Autodesk Inventor part; units mm, degrees
(part 2 of 3)
  measures "d37" diameter of A260
extrude "Extrusion3" add sketch "Sketch3" along normal blind 7.1 contours A0 | A211 | A196 L243 A245 | L243 A245 A196 | A159 | A208 | L220 A246 L224 A185 | A185 L224 A246 L220 | A206 | L219 A248 L216 A180 | A180 L216 A248 L219 | A151 | A153 | A189 | A207 | A213 | A218 | A221 | A222
extrude "Extrusion4" add sketch "Sketch3" along normal blind 2 contours A260 | A257 | A258 | A259
mirror "Mirror1" about plane through (0, 0, 0) normal (1, 0, 0) of "Extrusion4"
extrude "Extrusion5" add sketch "Sketch1" against normal up to surface (3 mm away) contours A10 L72 | L72 A10 | A75 | A27 | A76 | A77 L70 A15 L26 | L26 A15 L70 A77 | L26 L70 A15 | A15 L70 L26 | A78 L28 A12 L69 | L69 A12 L28 A78 | L69 L28 A12 | A12 L28 L69
mirror "Mirror2" about plane through (0, 0, 0) normal (1, 0, 0) of "Extrusion5"
sketch "Sketch4" plane through (0, 5, 0) normal (0, 1, 0) x (1, 0, 0)
  circle A0 centre (0, 0) radius 5.5
  dimension "d46" = 11
  constraints: 1 centre point, 1 coincident
  measures "d46" diameter of A0
extrude "Extrusion6" cut sketch "Sketch4" against normal blind 15
sketch "Sketch5" plane through (0, 5, 0) normal (0, 1, 0) x (1, 0, 0)
  arc A0 (19.2671, 3.2712) -> (23.1562, 4.8822) centre (19.2671, 8.7712) ccw projected
  line L0 (23.1562, 4.8822) -> (40.8632, 22.5892) projected
  circle A1 centre (17.1458, 27.8631) radius 5.5 projected
  circle A2 centre (17.1458, 27.8631) radius 5.5 projected
  arc A3 (23.1562, 4.8822) -> (19.2671, 3.2712) centre (19.2671, 8.7712) ccw projected
  line L1 (23.1562, 4.8822) -> (31.6415, 13.3674) projected
  circle A4 centre (27.7524, 17.2565) radius 5.5 projected
  circle A5 centre (27.7524, 17.2565) radius 5.5 projected
  line L2 (31.6415, 13.3674) -> (40.8632, 22.5892) projected
  line L3 (40.8632, 22.5892) -> (22.4784, 40.9739) projected
  line L4 (40.8632, 22.5892) -> (22.4784, 40.9739) projected
  line L5 (22.4784, 40.9739) -> (13.2567, 31.7522) projected
  line L6 (22.4784, 40.9739) -> (4.7714, 23.2669) projected
  circle A6 centre (8.6605, -19.0931) radius 2.5 projected
  circle A7 centre (8.6605, -19.0931) radius 1.5 projected
  circle A8 centre (19.2671, -8.4864) radius 1.5 projected
  circle A9 centre (19.2671, -8.4864) radius 1.5 projected
  circle A10 centre (19.2671, -8.4864) radius 1.5 projected
  circle A11 centre (19.2671, -8.4864) radius 2.5 projected
  circle A12 centre (19.2671, -8.4864) radius 2.5 projected
  circle A13 centre (19.2671, -8.4864) radius 2.5 projected
  circle A14 centre (19.2671, -8.4864) radius 3 projected
  circle A15 centre (19.2671, -8.4864) radius 5.5 projected
  circle A16 centre (19.2671, -8.4864) radius 3 projected
  circle A17 centre (19.2671, -8.4864) radius 3 projected
  circle A18 centre (19.2671, -8.4864) radius 2.5 projected
  circle A19 centre (19.2671, -8.4864) radius 3 projected
  circle A20 centre (19.2671, -8.4864) radius 3 projected
  circle A21 centre (8.6605, -19.0931) radius 1.5 projected
  circle A22 centre (8.6605, -19.0931) radius 1.5 projected
  circle A23 centre (8.6605, -19.0931) radius 1.5 projected
  circle A24 centre (8.6605, -19.0931) radius 1.5 projected
  circle A25 centre (8.6605, -19.0931) radius 2.5 projected
  circle A26 centre (8.6605, -19.0931) radius 1.5 projected
  circle A27 centre (8.6605, -19.0931) radius 2.5 projected
  circle A28 centre (8.6605, -19.0931) radius 2.5 projected
  circle A29 centre (8.6605, -19.0931) radius 2.5 projected
  circle A30 centre (8.6605, -19.0931) radius 3 projected
  circle A31 centre (8.6605, -19.0931) radius 3 projected
  circle A32 centre (8.6605, -19.0931) radius 2.5 projected
  circle A33 centre (8.6605, -19.0931) radius 3 projected
  circle A34 centre (8.6605, -19.0931) radius 3 projected
  circle A35 centre (8.6605, -19.0931) radius 3 projected
  circle A36 centre (8.6605, -19.0931) radius 5.5 projected
  circle A37 centre (8.6605, -19.0931) radius 5.5 projected
  arc A38 (3.1605, -19.0931) -> (4.7714, -22.9821) centre (8.6605, -19.0931) ccw projected
  arc A39 (4.7714, -22.9821) -> (3.1605, -19.0931) centre (8.6605, -19.0931) ccw projected
  line L7 (3.1605, -5.8386) -> (3.1605, -19.0931) projected
  line L8 (3.1605, -5.8386) -> (3.1605, -19.0931) projected
  circle A40 centre (19.2671, -8.4864) radius 1.5 projected
  arc A41 (23.1562, -4.5974) -> (19.2671, -2.9864) centre (19.2671, -8.4864) ccw projected
  line L9 (19.2671, -2.9864) -> (6.0127, -2.9864) projected
  arc A42 (6.0127, -2.9864) -> (6.0127, 3.2712) centre (0.0316, 0.1424) ccw projected
  line L10 (6.0127, 3.2712) -> (19.2671, 3.2712) projected
  arc A43 (3.1605, 6.1234) -> (-3.0972, 6.1234) centre (0.0316, 0.1424) ccw projected
  line L11 (6.0127, 3.2712) -> (19.2671, 3.2712) projected
  arc A44 (3.1605, 6.1234) -> (-3.0972, 6.1234) centre (0.0316, 0.1424) ccw projected
  arc A45 (3.1605, 6.1234) -> (-3.0972, 6.1234) centre (0.0316, 0.1424) ccw projected
  arc A46 (3.1605, 6.1234) -> (-3.0972, 6.1234) centre (0.0316, 0.1424) ccw projected
  arc A47 (6.0127, -2.9864) -> (6.0127, 3.2712) centre (0.0316, 0.1424) ccw projected
  line L12 (19.2671, -2.9864) -> (6.0127, -2.9864) projected
  arc A48 (6.0127, -2.9864) -> (6.0127, 3.2712) centre (0.0316, 0.1424) ccw projected
  arc A49 (6.0127, -2.9864) -> (6.0127, 3.2712) centre (0.0316, 0.1424) ccw projected
  arc A50 (19.2671, -2.9864) -> (23.1562, -4.5974) centre (19.2671, -8.4864) ccw projected
  arc A51 (-3.0972, -5.8386) -> (3.1605, -5.8386) centre (0.0316, 0.1424) ccw projected
  arc A52 (-3.0972, -5.8386) -> (3.1605, -5.8386) centre (0.0316, 0.1424) ccw projected
  circle A53 centre (0, 0) radius 5.5 projected
  line L13 (3.1605, -5.8386) -> (3.1605, -19.0931) projected
  arc A54 (3.1605, -19.0931) -> (4.7714, -22.9821) centre (8.6605, -19.0931) ccw projected
  line L14 (-3.0972, -19.0931) -> (-3.0972, -5.8386) projected
  circle A55 centre (0, 0) radius 5.5 projected
  circle A56 centre (17.1458, -27.5783) radius 2.5 projected
  circle A57 centre (17.1458, -27.5783) radius 1.5 projected
  circle A58 centre (17.1458, -27.5783) radius 1.5 projected
  circle A59 centre (17.1458, -27.5783) radius 2.5 projected
  circle A60 centre (17.1458, -27.5783) radius 3 projected
  line L15 (22.4651, -26.1801) -> (18.544, -22.259) projected
  line L16 (18.544, -22.259) -> (22.4651, -26.1801) projected
  arc A61 (18.544, -22.259) -> (13.2567, -31.4674) centre (17.1458, -27.5783) ccw projected
  arc A62 (18.544, -22.259) -> (22.4651, -26.1801) centre (17.1458, -27.5783) ccw projected
  arc A63 (13.2567, -31.4674) -> (22.4651, -26.1801) centre (17.1458, -27.5783) ccw projected
  circle A64 centre (17.1458, -27.5783) radius 3 projected
  line L17 (18.544, -22.259) -> (22.4651, -26.1801) projected
  arc A65 (18.544, -22.259) -> (22.4651, -26.1801) centre (17.1458, -27.5783) ccw projected
  circle A66 centre (17.1458, -27.5783) radius 1.5 projected
  circle A67 centre (17.1458, -27.5783) radius 1.5 projected
  circle A68 centre (17.1458, -27.5783) radius 1.5 projected
  circle A69 centre (17.1458, -27.5783) radius 2.5 projected
  circle A70 centre (17.1458, -27.5783) radius 2.5 projected
  circle A71 centre (17.1458, -27.5783) radius 3 projected
  circle A72 centre (17.1458, -27.5783) radius 3 projected
  circle A73 centre (17.1458, -27.5783) radius 3 projected
  circle A74 centre (17.1458, -27.5783) radius 2.5 projected
  circle A75 centre (17.1458, -27.5783) radius 2.5 projected
  circle A76 centre (17.1458, -27.5783) radius 1.5 projected
  line L18 (3.1605, -5.8386) -> (3.1605, -19.0931) projected
  arc A77 (4.7714, -22.9821) -> (3.1605, -19.0931) centre (8.6605, -19.0931) ccw projected
  line L19 (4.7714, -22.9821) -> (13.2567, -31.4674) projected
  line L20 (31.6415, -13.0826) -> (23.1562, -4.5974) projected
  circle A78 centre (19.2671, -8.4864) radius 5.5 projected
  line L21 (22.4651, -26.1801) -> (18.544, -22.259) projected
  line L22 (22.4331, -18.3699) -> (26.3542, -22.291) projected
  arc A79 (18.544, -22.259) -> (13.2567, -31.4674) centre (17.1458, -27.5783) ccw projected
  arc A80 (31.6415, -13.0826) -> (22.4331, -18.3699) centre (27.7524, -16.9717) ccw projected
  arc A81 (26.3542, -22.291) -> (31.6415, -13.0826) centre (27.7524, -16.9717) ccw projected
  arc A82 (13.2567, -31.4674) -> (22.4651, -26.1801) centre (17.1458, -27.5783) ccw projected
  circle A83 centre (8.6605, -19.0931) radius 5.5 projected
  arc A84 (4.7714, 23.2669) -> (3.1605, 19.3778) centre (8.6605, 19.3778) ccw projected
  line L23 (3.1605, 19.3778) -> (3.1605, 6.1234) projected
  line L24 (-3.0972, 6.1234) -> (-3.0972, 19.3778) projected
  arc A85 (-3.0972, 19.3778) -> (-4.7081, 23.2669) centre (-8.5972, 19.3778) ccw projected
  circle A86 centre (-8.5972, 19.3778) radius 1.5 projected
  circle A87 centre (-8.5972, 19.3778) radius 2.5 projected
  arc A88 (-8.6288, 16.878) -> (-8.6288, 21.8776) centre (-8.5972, 19.3778) ccw projected
  circle A89 centre (-8.6605, 19.3778) radius 3 projected
  arc A90 (-8.6288, 21.8776) -> (-8.6288, 16.878) centre (-8.6605, 19.3778) ccw projected
  arc A91 (-3.0972, -5.8386) -> (3.1605, -5.8386) centre (0.0316, 0.1424) ccw projected
  arc A92 (-3.0972, -5.8386) -> (3.1605, -5.8386) centre (0.0316, 0.1424) ccw projected
  circle A93 centre (-8.5972, 19.3778) radius 1.5 projected
  arc A94 (-8.6288, 21.8776) -> (-8.6288, 16.878) centre (-8.6605, 19.3778) ccw projected
  arc A95 (-8.6288, 21.8776) -> (-8.6288, 16.878) centre (-8.5972, 19.3778) ccw projected
  arc A96 (-8.6288, 21.8776) -> (-8.6288, 16.878) centre (-8.6605, 19.3778) ccw projected
  arc A97 (-8.6288, 21.8776) -> (-8.6288, 16.878) centre (-8.6605, 19.3778) ccw projected
  circle A98 centre (-8.5972, 19.3778) radius 5.5 projected
  circle A99 centre (-8.6605, 19.3778) radius 3 projected
  arc A100 (-8.6288, 16.878) -> (-8.6288, 21.8776) centre (-8.5972, 19.3778) ccw projected
  arc A101 (-8.6288, 21.8776) -> (-8.6288, 16.878) centre (-8.6605, 19.3778) ccw projected
  circle A102 centre (-8.6605, 19.3778) radius 3 projected
  circle A103 centre (-8.6605, 19.3778) radius 3 projected
  circle A104 centre (-8.6605, 19.3778) radius 3 projected
  circle A105 centre (-8.5972, 19.3778) radius 2.5 projected
  circle A106 centre (-8.5972, 19.3778) radius 1.5 projected
  arc A107 (-8.6288, 16.878) -> (-8.6288, 21.8776) centre (-8.5972, 19.3778) ccw projected
  arc A108 (-8.6288, 21.8776) -> (-8.6288, 16.878) centre (-8.5972, 19.3778) ccw projected
  circle A109 centre (-8.5972, 19.3778) radius 2.5 projected
  circle A110 centre (0, 0) radius 5.5 projected
  circle A111 centre (0, 0) radius 5.5 projected
  circle A112 centre (-8.5972, 19.3778) radius 1.5 projected
  circle A113 centre (-8.5972, 19.3778) radius 1.5 projected
  arc A114 (-19.2354, 11.271) -> (-19.2354, 6.2714) centre (-19.2038, 8.7712) ccw projected
  line L25 (13.2567, -31.4674) -> (22.4784, -40.6891) projected
  line L26 (22.4784, -40.6891) -> (40.8632, -22.3044) projected
  line L27 (40.8632, -22.3044) -> (31.6415, -13.0826) projected
  line L28 (4.7714, -22.9821) -> (22.4784, -40.6891) projected
  line L29 (22.4784, -40.6891) -> (40.8632, -22.3044) projected
  line L30 (40.8632, -22.3044) -> (23.1562, -4.5974) projected
  arc A115 (18.544, -22.259) -> (22.4651, -26.1801) centre (17.1458, -27.5783) ccw projected
  line L31 (18.544, -22.259) -> (22.4651, -26.1801) projected
  line L32 (26.3542, -22.291) -> (22.4331, -18.3699) projected
  arc A116 (26.3542, -22.291) -> (22.4331, -18.3699) centre (27.7524, -16.9717) ccw projected
  line L33 (19.2671, -2.9864) -> (6.0127, -2.9864) projected
  line L34 (19.2671, -2.9864) -> (6.0127, -2.9864) projected
  circle A117 centre (8.6605, -19.0931) radius 3 projected
  circle A118 centre (19.2671, -8.4864) radius 5.5 projected
  arc A119 (23.1562, -4.5974) -> (19.2671, -2.9864) centre (19.2671, -8.4864) ccw projected
  arc A120 (19.2671, -2.9864) -> (23.1562, -4.5974) centre (19.2671, -8.4864) ccw projected
  circle A121 centre (27.7524, -16.9717) radius 3 projected
  circle A122 centre (17.1458, -27.5783) radius 3 projected
  line L35 (4.7714, -22.9821) -> (13.2567, -31.4674) projected
  line L36 (13.2567, -31.4674) -> (22.4784, -40.6891) projected
  line L37 (4.7714, -22.9821) -> (22.4784, -40.6891) projected
  line L38 (40.8632, -22.3044) -> (31.6415, -13.0826) projected
  line L39 (31.6415, -13.0826) -> (23.1562, -4.5974) projected
  line L40 (40.8632, -22.3044) -> (23.1562, -4.5974) projected
  line L41 (22.4784, -40.6891) -> (40.8632, -22.3044) projected
  line L42 (22.4784, -40.6891) -> (40.8632, -22.3044) projected
  circle A123 centre (19.2671, -8.4864) radius 3 projected
  line L43 (13.2567, 31.7522) -> (4.7714, 23.2669) projected
  line L44 (3.1605, 19.3778) -> (3.1605, 6.1234) projected
  arc A124 (3.1605, 19.3778) -> (4.7714, 23.2669) centre (8.6605, 19.3778) ccw projected
  circle A125 centre (0, 0) radius 5.5 projected
  line L45 (4.7714, -22.9821) -> (22.4784, -40.6891) projected
  line L46 (22.4784, -40.6891) -> (40.8632, -22.3044) projected
  line L47 (40.8632, -22.3044) -> (23.1562, -4.5974) projected
  arc A126 (23.1562, -4.5974) -> (19.2671, -2.9864) centre (19.2671, -8.4864) ccw projected
  line L48 (19.2671, -2.9864) -> (6.0127, -2.9864) projected
  arc A127 (6.0127, -2.9864) -> (6.0127, 3.2712) centre (0.0316, 0.1424) ccw projected
  line L49 (6.0127, 3.2712) -> (19.2671, 3.2712) projected
  arc A128 (19.2671, 3.2712) -> (23.1562, 4.8822) centre (19.2671, 8.7712) ccw projected
  line L50 (23.1562, 4.8822) -> (40.8632, 22.5892) projected
  line L51 (40.8632, 22.5892) -> (22.4784, 40.9739) projected
  line L52 (22.4784, 40.9739) -> (4.7714, 23.2669) projected
  arc A129 (4.7714, 23.2669) -> (3.1605, 19.3778) centre (8.6605, 19.3778) ccw projected
  line L53 (3.1605, 19.3778) -> (3.1605, 6.1234) projected
  arc A130 (3.1605, 6.1234) -> (-3.0972, 6.1234) centre (0.0316, 0.1424) ccw projected
  line L54 (-3.0972, 6.1234) -> (-3.0972, 19.3778) projected
  arc A131 (-3.0972, 19.3778) -> (-4.7081, 23.2669) centre (-8.5972, 19.3778) ccw projected
  line L55 (-4.7081, 23.2669) -> (-22.4151, 40.9739) projected
  line L56 (-22.4151, 40.9739) -> (-40.7999, 22.5892) projected
  line L57 (-40.7999, 22.5892) -> (-23.0929, 4.8822) projected
  arc A132 (-23.0929, 4.8822) -> (-19.2038, 3.2712) centre (-19.2038, 8.7712) ccw projected
  line L58 (-19.2038, 3.2712) -> (-5.9494, 3.2712) projected
  arc A133 (-5.9494, 3.2712) -> (-5.9494, -2.9864) centre (0.0316, 0.1424) ccw projected
  line L59 (-5.9494, -2.9864) -> (-19.2038, -2.9864) projected
  arc A134 (-19.2038, -2.9864) -> (-23.0929, -4.5974) centre (-19.2038, -8.4864) ccw projected
  line L60 (-23.0929, -4.5974) -> (-40.7999, -22.3044) projected
  line L61 (-40.7999, -22.3044) -> (-22.4151, -40.6891) projected
  line L62 (-22.4151, -40.6891) -> (-4.7081, -22.9821) projected
  arc A135 (-4.7081, -22.9821) -> (-3.0972, -19.0931) centre (-8.5972, -19.0931) ccw projected
  line L63 (-3.0972, -19.0931) -> (-3.0972, -5.8386) projected
  arc A136 (-3.0972, -5.8386) -> (3.1605, -5.8386) centre (0.0316, 0.1424) ccw projected
  line L64 (3.1605, -5.8386) -> (3.1605, -19.0931) projected
  arc A137 (3.1605, -19.0931) -> (4.7714, -22.9821) centre (8.6605, -19.0931) ccw projected
  circle A138 centre (0, 0) radius 5.5 projected
  arc A139 (23.1562, 4.8822) -> (19.2671, 3.2712) centre (19.2671, 8.7712) ccw projected
  line L65 (6.0127, 3.2712) -> (19.2671, 3.2712) projected
  arc A140 (6.0127, -2.9864) -> (6.0127, 3.2712) centre (0.0316, 0.1424) ccw projected
  line L66 (19.2671, -2.9864) -> (6.0127, -2.9864) projected
  arc A141 (19.2671, -2.9864) -> (23.1562, -4.5974) centre (19.2671, -8.4864) ccw projected
  line L67 (31.6415, -13.0826) -> (23.1562, -4.5974) projected
  arc A142 (31.6415, -13.0826) -> (22.4331, -18.3699) centre (27.7524, -16.9717) ccw projected
  line L68 (22.4331, -18.3699) -> (26.3542, -22.291) projected
  arc A143 (26.3542, -22.291) -> (31.6415, -13.0826) centre (27.7524, -16.9717) ccw projected
  line L69 (40.8632, -22.3044) -> (31.6415, -13.0826) projected
  line L70 (22.4784, -40.6891) -> (40.8632, -22.3044) projected
  line L71 (13.2567, -31.4674) -> (22.4784, -40.6891) projected
  arc A144 (13.2567, -31.4674) -> (22.4651, -26.1801) centre (17.1458, -27.5783) ccw projected
  line L72 (22.4651, -26.1801) -> (18.544, -22.259) projected
  arc A145 (18.544, -22.259) -> (13.2567, -31.4674) centre (17.1458, -27.5783) ccw projected
  line L73 (4.7714, -22.9821) -> (13.2567, -31.4674) projected
  arc A146 (4.7714, -22.9821) -> (3.1605, -19.0931) centre (8.6605, -19.0931) ccw projected
  line L74 (3.1605, -5.8386) -> (3.1605, -19.0931) projected
  arc A147 (-3.0972, -5.8386) -> (3.1605, -5.8386) centre (0.0316, 0.1424) ccw projected
  line L75 (-3.0972, -19.0931) -> (-3.0972, -5.8386) projected
  arc A148 (-3.0972, -19.0931) -> (-4.7081, -22.9821) centre (-8.5972, -19.0931) ccw projected
  line L76 (-13.1934, -31.4674) -> (-4.7081, -22.9821) projected
  circle A149 centre (-17.0825, -27.5783) radius 5.5 projected
  line L77 (-22.4151, -40.6891) -> (-13.1934, -31.4674) projected
  line L78 (-40.7999, -22.3044) -> (-22.4151, -40.6891) projected
  line L79 (-31.5782, -13.0826) -> (-40.7999, -22.3044) projected
  circle A150 centre (-27.6891, -16.9717) radius 5.5 projected
  line L80 (-23.0929, -4.5974) -> (-31.5782, -13.0826) projected
  arc A151 (-23.0929, -4.5974) -> (-19.2038, -2.9864) centre (-19.2038, -8.4864) ccw projected
  line L81 (-5.9494, -2.9864) -> (-19.2038, -2.9864) projected
  arc A152 (-5.9494, 3.2712) -> (-5.9494, -2.9864) centre (0.0316, 0.1424) ccw projected
  line L82 (-19.2038, 3.2712) -> (-5.9494, 3.2712) projected
  arc A153 (-19.2038, 3.2712) -> (-23.0929, 4.8822) centre (-19.2038, 8.7712) ccw projected
  line L83 (-31.5782, 13.3674) -> (-23.0929, 4.8822) projected
  circle A154 centre (-27.6891, 17.2565) radius 5.5 projected
  line L84 (-40.7999, 22.5892) -> (-31.5782, 13.3674) projected
  line L85 (-22.4151, 40.9739) -> (-40.7999, 22.5892) projected
  line L86 (-13.1934, 31.7522) -> (-22.4151, 40.9739) projected
  circle A155 centre (-17.0825, 27.8631) radius 5.5 projected
  line L87 (-4.7081, 23.2669) -> (-13.1934, 31.7522) projected
  arc A156 (-4.7081, 23.2669) -> (-3.0972, 19.3778) centre (-8.5972, 19.3778) ccw projected
  line L88 (-3.0972, 6.1234) -> (-3.0972, 19.3778) projected
  arc A157 (3.1605, 6.1234) -> (-3.0972, 6.1234) centre (0.0316, 0.1424) ccw projected
  line L89 (3.1605, 19.3778) -> (3.1605, 6.1234) projected
  arc A158 (3.1605, 19.3778) -> (4.7714, 23.2669) centre (8.6605, 19.3778) ccw projected
  line L90 (13.2567, 31.7522) -> (4.7714, 23.2669) projected
  circle A159 centre (17.1458, 27.8631) radius 5.5 projected
  line L91 (22.4784, 40.9739) -> (13.2567, 31.7522) projected
  line L92 (40.8632, 22.5892) -> (22.4784, 40.9739) projected
  line L93 (31.6415, 13.3674) -> (40.8632, 22.5892) projected
  circle A160 centre (27.7524, 17.2565) radius 5.5 projected
  line L94 (23.1562, 4.8822) -> (31.6415, 13.3674) projected
  arc A161 (-4.7081, -22.9821) -> (-3.0972, -19.0931) centre (-8.5972, -19.0931) ccw projected
  arc A162 (-5.9494, 3.2712) -> (-5.9494, -2.9864) centre (0.0316, 0.1424) ccw projected
  line L95 (-4.7081, 23.2669) -> (-22.4151, 40.9739) projected
  arc A163 (-23.0929, 4.8822) -> (-19.2038, 3.2712) centre (-19.2038, 8.7712) ccw projected
  line L96 (-5.9494, -2.9864) -> (-19.2038, -2.9864) projected
  arc A164 (-19.2038, -2.9864) -> (-23.0929, -4.5974) centre (-19.2038, -8.4864) ccw projected
  line L97 (-22.4151, 40.9739) -> (-40.7999, 22.5892) projected
  line L98 (-40.7999, 22.5892) -> (-23.0929, 4.8822) projected
  line L99 (-19.2038, 3.2712) -> (-5.9494, 3.2712) projected
  arc A165 (-4.7081, 23.2669) -> (-3.0972, 19.3778) centre (-8.5972, 19.3778) ccw projected
  line L100 (-4.7081, 23.2669) -> (-13.1934, 31.7522) projected
  circle A166 centre (-19.2038, 8.7712) radius 1.5 projected
  circle A167 centre (-8.5972, 19.3778) radius 1.5 projected
  circle A168 centre (-19.2671, 8.7712) radius 3 projected
  circle A169 centre (-8.6605, 19.3778) radius 3 projected
  circle A170 centre (-8.5972, 19.3778) radius 5.5 projected
  circle A171 centre (-19.2038, 8.7712) radius 5.5 projected
  circle A172 centre (-17.0825, 27.8631) radius 1.5 projected
  circle A173 centre (-17.0825, 27.8631) radius 5.5 projected
  circle A174 centre (-27.8428, 17.2565) radius 1.5 projected
  arc A175 (-19.2354, 11.271) -> (-19.2354, 6.2714) centre (-19.2671, 8.7712) ccw projected
  circle A176 centre (-27.8428, 17.2565) radius 1.5 projected
  circle A177 centre (-17.0825, 27.8631) radius 1.5 projected
  circle A178 centre (-17.0825, 27.8631) radius 2.5 projected
  arc A179 (-17.1141, 30.3629) -> (-17.1141, 25.3633) centre (-17.0825, 27.8631) ccw projected
  circle A180 centre (-27.6891, 17.2565) radius 2.5 projected
  arc A181 (-27.7207, 19.7563) -> (-27.7207, 14.7567) centre (-27.6891, 17.2565) ccw projected
  arc A182 (-17.1141, 25.3633) -> (-17.1141, 30.3629) centre (-17.0825, 27.8631) ccw projected
  circle A183 centre (-17.1458, 27.8631) radius 3 projected
  circle A184 centre (-17.1458, 27.8631) radius 3 projected
  arc A185 (-17.1141, 30.3629) -> (-17.1141, 25.3633) centre (-17.1458, 27.8631) ccw projected
  arc A186 (-17.1141, 30.3629) -> (-17.1141, 25.3633) centre (-17.1458, 27.8631) ccw projected
  arc A187 (-27.7207, 14.7567) -> (-27.7207, 19.7563) centre (-27.6891, 17.2565) ccw projected
  circle A188 centre (-27.8428, 17.2565) radius 1.5 projected
  circle A189 centre (-27.8428, 17.2565) radius 1.5 projected
  circle A190 centre (-27.8428, 17.2565) radius 1.5 projected
  arc A191 (-17.1141, 30.3629) -> (-17.1141, 25.3633) centre (-17.1458, 27.8631) ccw projected
  arc A192 (-17.1141, 30.3629) -> (-17.1141, 25.3633) centre (-17.1458, 27.8631) ccw projected
  arc A193 (-17.1141, 30.3629) -> (-17.1141, 25.3633) centre (-17.1458, 27.8631) ccw projected
  arc A194 (-17.1141, 30.3629) -> (-17.1141, 25.3633) centre (-17.0825, 27.8631) ccw projected
  circle A195 centre (-17.0825, 27.8631) radius 1.5 projected
  circle A196 centre (-17.0825, 27.8631) radius 1.5 projected
  circle A197 centre (-17.0825, 27.8631) radius 1.5 projected
  arc A198 (-17.1141, 25.3633) -> (-17.1141, 30.3629) centre (-17.0825, 27.8631) ccw projected
  arc A199 (-17.1141, 30.3629) -> (-17.1141, 25.3633) centre (-17.1458, 27.8631) ccw projected
  circle A200 centre (-17.1458, 27.8631) radius 3 projected
  circle A201 centre (-17.1458, 27.8631) radius 3 projected
  circle A202 centre (-17.1458, 27.8631) radius 3 projected
  circle A203 centre (-17.0825, 27.8631) radius 5.5 projected
  circle A204 centre (-17.0825, 27.8631) radius 5.5 projected
  circle A205 centre (-17.0825, 27.8631) radius 5.5 projected
  circle A206 centre (-17.1458, 27.8631) radius 3 projected
  circle A207 centre (-17.0825, 27.8631) radius 2.5 projected
  circle A208 centre (-17.0825, 27.8631) radius 1.5 projected
  arc A209 (-17.1141, 25.3633) -> (-17.1141, 30.3629) centre (-17.0825, 27.8631) ccw projected
  arc A210 (-17.1141, 30.3629) -> (-17.1141, 25.3633) centre (-17.0825, 27.8631) ccw projected
  circle A211 centre (-17.0825, 27.8631) radius 2.5 projected
  arc A212 (-27.7207, 14.7567) -> (-27.7207, 19.7563) centre (-27.6891, 17.2565) ccw projected
  arc A213 (-27.7207, 19.7563) -> (-27.7207, 14.7567) centre (-27.6891, 17.2565) ccw projected
  circle A214 centre (-27.6891, 17.2565) radius 2.5 projected
  line L101 (-13.1934, 31.7522) -> (-22.4151, 40.9739) projected
  line L102 (-22.4151, 40.9739) -> (-40.7999, 22.5892) projected
  line L103 (-40.7999, 22.5892) -> (-31.5782, 13.3674) projected
  line L104 (-19.2038, 3.2712) -> (-5.9494, 3.2712) projected
  line L105 (-19.2038, 3.2712) -> (-5.9494, 3.2712) projected
  line L106 (-3.0972, 6.1234) -> (-3.0972, 19.3778) projected
  line L107 (-3.0972, 6.1234) -> (-3.0972, 19.3778) projected
  circle A215 centre (-19.2038, 8.7712) radius 5.5 projected
  arc A216 (-23.0929, 4.8822) -> (-19.2038, 3.2712) centre (-19.2038, 8.7712) ccw projected
  arc A217 (-19.2038, 3.2712) -> (-23.0929, 4.8822) centre (-19.2038, 8.7712) ccw projected
  circle A218 centre (-8.5972, 19.3778) radius 5.5 projected
  arc A219 (-3.0972, 19.3778) -> (-4.7081, 23.2669) centre (-8.5972, 19.3778) ccw projected
  arc A220 (-4.7081, 23.2669) -> (-3.0972, 19.3778) centre (-8.5972, 19.3778) ccw projected
  circle A221 centre (-27.7524, 17.2565) radius 3 projected
  line L108 (-4.7081, 23.2669) -> (-13.1934, 31.7522) projected
  line L109 (-13.1934, 31.7522) -> (-22.4151, 40.9739) projected
  line L110 (-4.7081, 23.2669) -> (-22.4151, 40.9739) projected
  line L111 (-40.7999, 22.5892) -> (-31.5782, 13.3674) projected
  line L112 (-31.5782, 13.3674) -> (-23.0929, 4.8822) projected
  line L113 (-40.7999, 22.5892) -> (-23.0929, 4.8822) projected
  line L114 (-22.4151, 40.9739) -> (-40.7999, 22.5892) projected
  line L115 (-22.4151, 40.9739) -> (-40.7999, 22.5892) projected
  arc A222 (-27.7207, 19.7563) -> (-27.7207, 14.7567) centre (-27.7524, 17.2565) ccw projected
  arc A223 (-8.6288, 21.8776) -> (-8.6288, 16.878) centre (-8.6605, 19.3778) ccw projected
  circle A224 centre (-27.6891, 17.2565) radius 5.5 projected
  circle A225 centre (-17.0825, 27.8631) radius 5.5 projected
  arc A226 (-8.6288, 21.8776) -> (-8.6288, 16.878) centre (-8.5972, 19.3778) ccw projected
  circle A227 centre (-27.6891, 17.2565) radius 2.5 projected
  circle A228 centre (-27.8428, 17.2565) radius 1.5 projected
  circle A229 centre (-19.2038, 8.7712) radius 1.5 projected
  circle A230 centre (-19.2038, 8.7712) radius 2.5 projected
  arc A231 (-19.2354, 6.2714) -> (-19.2354, 11.271) centre (-19.2038, 8.7712) ccw projected
  circle A232 centre (-19.2671, 8.7712) radius 3 projected
  arc A233 (-19.2354, 11.271) -> (-19.2354, 6.2714) centre (-19.2671, 8.7712) ccw projected
  arc A234 (-27.7207, 19.7563) -> (-27.7207, 14.7567) centre (-27.7524, 17.2565) ccw projected
  arc A235 (-27.7207, 19.7563) -> (-27.7207, 14.7567) centre (-27.6891, 17.2565) ccw projected
  arc A236 (-27.7207, 19.7563) -> (-27.7207, 14.7567) centre (-27.7524, 17.2565) ccw projected
  arc A237 (-27.7207, 19.7563) -> (-27.7207, 14.7567) centre (-27.7524, 17.2565) ccw projected
  circle A238 centre (-27.7524, 17.2565) radius 3 projected
  arc A239 (-27.7207, 14.7567) -> (-27.7207, 19.7563) centre (-27.6891, 17.2565) ccw projected
  arc A240 (-27.7207, 19.7563) -> (-27.7207, 14.7567) centre (-27.7524, 17.2565) ccw projected
  circle A241 centre (-27.7524, 17.2565) radius 3 projected
  circle A242 centre (-27.7524, 17.2565) radius 3 projected
  circle A243 centre (-27.7524, 17.2565) radius 3 projected
  circle A244 centre (-27.6891, 17.2565) radius 5.5 projected
  circle A245 centre (-27.6891, 17.2565) radius 5.5 projected
  circle A246 centre (-27.6891, 17.2565) radius 5.5 projected
  circle A247 centre (-27.7524, 17.2565) radius 3 projected
  circle A248 centre (-19.2038, 8.7712) radius 1.5 projected
  circle A249 centre (-19.2038, 8.7712) radius 1.5 projected
  circle A250 centre (-19.2038, 8.7712) radius 1.5 projected
  circle A251 centre (-19.2038, 8.7712) radius 2.5 projected
  circle A252 centre (-19.2038, 8.7712) radius 1.5 projected
  arc A253 (-19.2354, 6.2714) -> (-19.2354, 11.271) centre (-19.2038, 8.7712) ccw projected
  arc A254 (-19.2354, 11.271) -> (-19.2354, 6.2714) centre (-19.2038, 8.7712) ccw projected
  circle A255 centre (-19.2038, 8.7712) radius 2.5 projected
  circle A256 centre (-19.2038, 8.7712) radius 5.5 projected
  circle A257 centre (-19.2671, 8.7712) radius 3 projected
  arc A258 (-19.2354, 6.2714) -> (-19.2354, 11.271) centre (-19.2038, 8.7712) ccw projected
  arc A259 (-19.2354, 11.271) -> (-19.2354, 6.2714) centre (-19.2671, 8.7712) ccw projected
  circle A260 centre (-19.2671, 8.7712) radius 3 projected
  circle A261 centre (-19.2671, 8.7712) radius 3 projected
  circle A262 centre (-19.2671, 8.7712) radius 3 projected
  arc A263 (-19.2354, 11.271) -> (-19.2354, 6.2714) centre (-19.2671, 8.7712) ccw projected
  arc A264 (-19.2354, 11.271) -> (-19.2354, 6.2714) centre (-19.2038, 8.7712) ccw projected
  arc A265 (-19.2354, 11.271) -> (-19.2354, 6.2714) centre (-19.2671, 8.7712) ccw projected
  arc A266 (-19.2354, 11.271) -> (-19.2354, 6.2714) centre (-19.2671, 8.7712) ccw projected
  arc A267 (-27.7207, 19.7563) -> (-27.7207, 14.7567) centre (-27.7524, 17.2565) ccw projected
  circle A268 centre (-19.2038, -8.4864) radius 2.5 projected
  circle A269 centre (-19.2038, -8.4864) radius 1.5 projected
  circle A270 centre (-8.5972, -19.0931) radius 2.5 projected
  circle A271 centre (-8.5972, -19.0931) radius 1.5 projected
  circle A272 centre (-19.2671, -8.4864) radius 3 projected
  circle A273 centre (-19.2038, -8.4864) radius 1.5 projected
  circle A274 centre (-19.2038, -8.4864) radius 2.5 projected
  circle A275 centre (-19.2038, -8.4864) radius 1.5 projected
  circle A276 centre (-19.2038, -8.4864) radius 1.5 projected
  circle A277 centre (-19.2038, -8.4864) radius 1.5 projected
  circle A278 centre (-19.2671, -8.4864) radius 3 projected
  circle A279 centre (-19.2038, -8.4864) radius 5.5 projected
  circle A280 centre (-19.2671, -8.4864) radius 3 projected
  circle A281 centre (-19.2671, -8.4864) radius 3 projected
  circle A282 centre (-19.2038, -8.4864) radius 2.5 projected
  circle A283 centre (-19.2671, -8.4864) radius 3 projected
  circle A284 centre (-19.2671, -8.4864) radius 3 projected
  circle A285 centre (-19.2038, -8.4864) radius 2.5 projected
  circle A286 centre (-19.2038, -8.4864) radius 1.5 projected
  circle A287 centre (-19.2038, -8.4864) radius 2.5 projected
  circle A288 centre (-19.2038, -8.4864) radius 2.5 projected
  circle A289 centre (-8.5972, -19.0931) radius 1.5 projected
  circle A290 centre (-8.5972, -19.0931) radius 1.5 projected
  circle A291 centre (-8.5972, -19.0931) radius 2.5 projected
  circle A292 centre (-8.5972, -19.0931) radius 1.5 projected
  circle A293 centre (-8.5972, -19.0931) radius 2.5 projected
  circle A294 centre (-8.5972, -19.0931) radius 2.5 projected
  circle A295 centre (-8.5972, -19.0931) radius 1.5 projected
  circle A296 centre (-8.5972, -19.0931) radius 1.5 projected
  circle A297 centre (-8.5972, -19.0931) radius 2.5 projected
  circle A298 centre (-8.6605, -19.0931) radius 3 projected
  circle A299 centre (-8.6605, -19.0931) radius 3 projected
  circle A300 centre (-8.6605, -19.0931) radius 3 projected
  circle A301 centre (-8.6605, -19.0931) radius 3 projected
  line L116 (-3.0972, -19.0931) -> (-3.0972, -5.8386) projected
  line L117 (-3.0972, -19.0931) -> (-3.0972, -5.8386) projected
  circle A302 centre (-8.5972, -19.0931) radius 5.5 projected
  arc A303 (-4.7081, -22.9821) -> (-3.0972, -19.0931) centre (-8.5972, -19.0931) ccw projected
  arc A304 (-3.0972, -19.0931) -> (-4.7081, -22.9821) centre (-8.5972, -19.0931) ccw projected
  circle A305 centre (-8.6605, -19.0931) radius 3 projected
  circle A306 centre (-8.5972, -19.0931) radius 5.5 projected
  circle A307 centre (-8.6605, -19.0931) radius 3 projected
  circle A308 centre (-8.5972, -19.0931) radius 2.5 projected
  circle A309 centre (-17.0825, -27.5783) radius 2.5 projected
  circle A310 centre (-17.0825, -27.5783) radius 1.5 projected
  circle A311 centre (-17.0825, -27.5783) radius 1.5 projected
  circle A312 centre (-17.0825, -27.5783) radius 2.5 projected
  circle A313 centre (-17.0825, -27.5783) radius 1.5 projected
  circle A314 centre (-17.0825, -27.5783) radius 1.5 projected
  circle A315 centre (-17.0825, -27.5783) radius 2.5 projected
  circle A316 centre (-17.0825, -27.5783) radius 1.5 projected
  circle A317 centre (-17.0825, -27.5783) radius 2.5 projected
  circle A318 centre (-17.0825, -27.5783) radius 2.5 projected
  circle A319 centre (-17.1458, -27.5783) radius 3 projected
  circle A320 centre (-17.1458, -27.5783) radius 3 projected
  circle A321 centre (-17.0825, -27.5783) radius 2.5 projected
  circle A322 centre (-17.1458, -27.5783) radius 3 projected
  circle A323 centre (-17.1458, -27.5783) radius 3 projected
  circle A324 centre (-17.1458, -27.5783) radius 3 projected
  circle A325 centre (-17.0825, -27.5783) radius 5.5 projected
  circle A326 centre (-17.0825, -27.5783) radius 5.5 projected
  circle A327 centre (-17.0825, -27.5783) radius 5.5 projected
  circle A328 centre (-17.0825, -27.5783) radius 1.5 projected
  circle A329 centre (-27.6891, -16.9717) radius 2.5 projected
  circle A330 centre (-27.6891, -16.9717) radius 1.5 projected
  circle A331 centre (-27.6891, -16.9717) radius 1.5 projected
  circle A332 centre (-27.6891, -16.9717) radius 1.5 projected
  circle A333 centre (-27.6891, -16.9717) radius 2.5 projected
  circle A334 centre (-27.7524, -16.9717) radius 3 projected
  circle A335 centre (-27.7524, -16.9717) radius 3 projected
  circle A336 centre (-27.7524, -16.9717) radius 3 projected
  circle A337 centre (-27.7524, -16.9717) radius 3 projected
  circle A338 centre (-27.7524, -16.9717) radius 3 projected
  circle A339 centre (-27.6891, -16.9717) radius 2.5 projected
  circle A340 centre (-27.6891, -16.9717) radius 1.5 projected
  circle A341 centre (-27.6891, -16.9717) radius 1.5 projected
  circle A342 centre (-27.6891, -16.9717) radius 2.5 projected
  circle A343 centre (-27.6891, -16.9717) radius 2.5 projected
  circle A344 centre (-27.6891, -16.9717) radius 2.5 projected
  circle A345 centre (-27.6891, -16.9717) radius 1.5 projected
  circle A346 centre (-27.6891, -16.9717) radius 5.5 projected
  circle A347 centre (-27.6891, -16.9717) radius 5.5 projected
  circle A348 centre (-27.7524, -16.9717) radius 3 projected
  circle A349 centre (-27.6891, -16.9717) radius 5.5 projected
  line L118 (-3.0972, 6.1234) -> (-3.0972, 19.3778) projected
  line L119 (-31.5782, 13.3674) -> (-23.0929, 4.8822) projected
  arc A350 (-19.2038, 3.2712) -> (-23.0929, 4.8822) centre (-19.2038, 8.7712) ccw projected
  line L120 (-19.2038, 3.2712) -> (-5.9494, 3.2712) projected
  arc A351 (-5.9494, 3.2712) -> (-5.9494, -2.9864) centre (0.0316, 0.1424) ccw projected
  line L121 (-5.9494, -2.9864) -> (-19.2038, -2.9864) projected
  arc A352 (-23.0929, -4.5974) -> (-19.2038, -2.9864) centre (-19.2038, -8.4864) ccw projected
  line L122 (-23.0929, -4.5974) -> (-31.5782, -13.0826) projected
  line L123 (-3.0972, -19.0931) -> (-3.0972, -5.8386) projected
  arc A353 (-5.9494, 3.2712) -> (-5.9494, -2.9864) centre (0.0316, 0.1424) ccw projected
  arc A354 (-5.9494, 3.2712) -> (-5.9494, -2.9864) centre (0.0316, 0.1424) ccw projected
  arc A355 (-3.0972, -19.0931) -> (-4.7081, -22.9821) centre (-8.5972, -19.0931) ccw projected
  circle A356 centre (-8.5972, -19.0931) radius 5.5 projected
  line L124 (-13.1934, -31.4674) -> (-4.7081, -22.9821) projected
  line L125 (-22.4151, -40.6891) -> (-13.1934, -31.4674) projected
  circle A357 centre (-17.0825, -27.5783) radius 5.5 projected
  circle A358 centre (-17.0825, -27.5783) radius 5.5 projected
  line L126 (-40.7999, -22.3044) -> (-22.4151, -40.6891) projected
  circle A359 centre (-19.2038, -8.4864) radius 5.5 projected
  circle A360 centre (-27.6891, -16.9717) radius 5.5 projected
  circle A361 centre (-27.6891, -16.9717) radius 5.5 projected
  circle A362 centre (-27.6891, 17.2565) radius 5.5 projected
  line L127 (-5.9494, -2.9864) -> (-19.2038, -2.9864) projected
  line L128 (-5.9494, -2.9864) -> (-19.2038, -2.9864) projected
  line L129 (-22.4151, -40.6891) -> (-4.7081, -22.9821) projected
  line L130 (-31.5782, -13.0826) -> (-40.7999, -22.3044) projected
  circle A363 centre (-19.2038, -8.4864) radius 5.5 projected
  arc A364 (-19.2038, -2.9864) -> (-23.0929, -4.5974) centre (-19.2038, -8.4864) ccw projected
  arc A365 (-23.0929, -4.5974) -> (-19.2038, -2.9864) centre (-19.2038, -8.4864) ccw projected
  circle A366 centre (-17.1458, -27.5783) radius 3 projected
  line L131 (-23.0929, -4.5974) -> (-31.5782, -13.0826) projected
  line L132 (-31.5782, -13.0826) -> (-40.7999, -22.3044) projected
  line L133 (-23.0929, -4.5974) -> (-40.7999, -22.3044) projected
  line L134 (-22.4151, -40.6891) -> (-13.1934, -31.4674) projected
  line L135 (-13.1934, -31.4674) -> (-4.7081, -22.9821) projected
  line L136 (-22.4151, -40.6891) -> (-4.7081, -22.9821) projected
  line L137 (-40.7999, -22.3044) -> (-22.4151, -40.6891) projected
  line L138 (-40.7999, -22.3044) -> (-22.4151, -40.6891) projected
  line L139 (-40.7999, -22.3044) -> (-22.4151, -40.6891) projected
  line L140 (-23.0929, -4.5974) -> (-40.7999, -22.3044) projected
  circle A367 centre (19.2671, 8.7712) radius 1.5 projected
  circle A368 centre (27.7524, -16.9717) radius 2.5 projected
  circle A369 centre (27.7524, -16.9717) radius 1.5 projected
  line L141 (22.4331, -18.3699) -> (26.3542, -22.291) projected
  line L142 (26.3542, -22.291) -> (22.4331, -18.3699) projected
  circle A370 centre (27.7524, -16.9717) radius 1.5 projected
  circle A371 centre (27.7524, -16.9717) radius 1.5 projected
  circle A372 centre (27.7524, -16.9717) radius 2.5 projected
  circle A373 centre (27.7524, -16.9717) radius 1.5 projected
  circle A374 centre (27.7524, -16.9717) radius 2.5 projected
  circle A375 centre (27.7524, -16.9717) radius 2.5 projected
  circle A376 centre (27.7524, -16.9717) radius 1.5 projected
  circle A377 centre (27.7524, -16.9717) radius 1.5 projected
  circle A378 centre (27.7524, -16.9717) radius 2.5 projected
  arc A379 (26.3542, -22.291) -> (31.6415, -13.0826) centre (27.7524, -16.9717) ccw projected
  arc A380 (26.3542, -22.291) -> (22.4331, -18.3699) centre (27.7524, -16.9717) ccw projected
  arc A381 (31.6415, -13.0826) -> (22.4331, -18.3699) centre (27.7524, -16.9717) ccw projected
  circle A382 centre (27.7524, -16.9717) radius 3 projected
  arc A383 (26.3542, -22.291) -> (22.4331, -18.3699) centre (27.7524, -16.9717) ccw projected
  line L143 (26.3542, -22.291) -> (22.4331, -18.3699) projected
  circle A384 centre (27.7524, -16.9717) radius 3 projected
  circle A385 centre (27.7524, -16.9717) radius 3 projected
  circle A386 centre (27.7524, -16.9717) radius 2.5 projected
  circle A387 centre (27.7524, -16.9717) radius 3 projected
  circle A388 centre (27.7524, -16.9717) radius 3 projected
  circle A389 centre (19.2671, 8.7712) radius 1.5 projected
  circle A390 centre (19.2671, 8.7712) radius 3 projected
  circle A391 centre (19.2671, 8.7712) radius 5.5 projected
  circle A392 centre (27.7524, 17.2565) radius 3 projected
  circle A393 centre (27.7524, 17.2565) radius 2.5 projected
  circle A394 centre (17.1458, 27.8631) radius 1.5 projected
  circle A395 centre (17.1458, 27.8631) radius 3 projected
  circle A396 centre (17.1458, 27.8631) radius 5.5 projected
  circle A397 centre (27.7524, 17.2565) radius 2.5 projected
  circle A398 centre (19.2671, 8.7712) radius 2.5 projected
  circle A399 centre (19.2671, 8.7712) radius 1.5 projected
  circle A400 centre (27.7524, 17.2565) radius 1.5 projected
  circle A401 centre (27.7524, 17.2565) radius 2.5 projected
  circle A402 centre (27.7524, 17.2565) radius 1.5 projected
  circle A403 centre (27.7524, 17.2565) radius 2.5 projected
  circle A404 centre (27.7524, 17.2565) radius 2.5 projected
  circle A405 centre (19.2671, 8.7712) radius 1.5 projected
  circle A406 centre (19.2671, 8.7712) radius 1.5 projected
  circle A407 centre (19.2671, 8.7712) radius 2.5 projected
  circle A408 centre (19.2671, 8.7712) radius 2.5 projected
  circle A409 centre (19.2671, 8.7712) radius 2.5 projected
  circle A410 centre (19.2671, 8.7712) radius 1.5 projected
  circle A411 centre (19.2671, 8.7712) radius 3 projected
  circle A412 centre (19.2671, 8.7712) radius 3 projected
  circle A413 centre (19.2671, 8.7712) radius 2.5 projected
  circle A414 centre (19.2671, 8.7712) radius 3 projected
  circle A415 centre (19.2671, 8.7712) radius 3 projected
  circle A416 centre (19.2671, 8.7712) radius 2.5 projected
  circle A417 centre (27.7524, 17.2565) radius 3 projected
  circle A418 centre (27.7524, 17.2565) radius 3 projected
  circle A419 centre (27.7524, 17.2565) radius 3 projected
  circle A420 centre (27.7524, 17.2565) radius 5.5 projected
  circle A421 centre (27.7524, 17.2565) radius 5.5 projected
  circle A422 centre (27.7524, 17.2565) radius 3 projected
  circle A423 centre (27.7524, 17.2565) radius 5.5 projected
  circle A424 centre (27.7524, 17.2565) radius 2.5 projected
  circle A425 centre (27.7524, 17.2565) radius 1.5 projected
  circle A426 centre (27.7524, 17.2565) radius 1.5 projected
  circle A427 centre (17.1458, 27.8631) radius 2.5 projected
  circle A428 centre (17.1458, 27.8631) radius 1.5 projected
  circle A429 centre (17.1458, 27.8631) radius 1.5 projected
  circle A430 centre (8.6605, 19.3778) radius 2.5 projected
  circle A431 centre (8.6605, 19.3778) radius 1.5 projected
  circle A432 centre (8.6605, 19.3778) radius 1.5 projected
  circle A433 centre (17.1458, 27.8631) radius 1.5 projected
  circle A434 centre (17.1458, 27.8631) radius 1.5 projected
  circle A435 centre (17.1458, 27.8631) radius 2.5 projected
  circle A436 centre (17.1458, 27.8631) radius 2.5 projected
  circle A437 centre (17.1458, 27.8631) radius 1.5 projected
  circle A438 centre (17.1458, 27.8631) radius 2.5 projected
  circle A439 centre (17.1458, 27.8631) radius 2.5 projected
  circle A440 centre (17.1458, 27.8631) radius 3 projected
  circle A441 centre (17.1458, 27.8631) radius 3 projected
  circle A442 centre (17.1458, 27.8631) radius 2.5 projected
  circle A443 centre (17.1458, 27.8631) radius 3 projected
  circle A444 centre (17.1458, 27.8631) radius 3 projected
  circle A445 centre (17.1458, 27.8631) radius 5.5 projected
  circle A446 centre (17.1458, 27.8631) radius 5.5 projected
  circle A447 centre (8.6605, 19.3778) radius 1.5 projected
  circle A448 centre (8.6605, 19.3778) radius 2.5 projected
  circle A449 centre (8.6605, 19.3778) radius 3 projected
  circle A450 centre (8.6605, 19.3778) radius 5.5 projected
  circle A451 centre (8.6605, 19.3778) radius 3 projected
  circle A452 centre (8.6605, 19.3778) radius 3 projected
  circle A453 centre (8.6605, 19.3778) radius 2.5 projected
  circle A454 centre (8.6605, 19.3778) radius 3 projected
  circle A455 centre (8.6605, 19.3778) radius 3 projected
  circle A456 centre (8.6605, 19.3778) radius 2.5 projected
  circle A457 centre (8.6605, 19.3778) radius 1.5 projected
  circle A458 centre (8.6605, 19.3778) radius 2.5 projected
  circle A459 centre (8.6605, 19.3778) radius 2.5 projected
  circle A460 centre (8.6605, 19.3778) radius 1.5 projected
  circle A461 centre (8.6605, 19.3778) radius 1.5 projected
  circle A462 centre (27.7524, 17.2565) radius 1.5 projected
  circle A463 centre (27.7524, 17.2565) radius 1.5 projected
  circle A464 centre (8.6605, 19.3778) radius 3 projected
  line L144 (6.0127, 3.2712) -> (19.2671, 3.2712) projected
  line L145 (6.0127, 3.2712) -> (19.2671, 3.2712) projected
  circle A465 centre (8.6605, 19.3778) radius 5.5 projected
  circle A466 centre (8.6605, 19.3778) radius 5.5 projected
  arc A467 (4.7714, 23.2669) -> (3.1605, 19.3778) centre (8.6605, 19.3778) ccw projected
  arc A468 (3.1605, 19.3778) -> (4.7714, 23.2669) centre (8.6605, 19.3778) ccw projected
  circle A469 centre (19.2671, 8.7712) radius 3 projected
  circle A470 centre (19.2671, 8.7712) radius 5.5 projected
  arc A471 (19.2671, 3.2712) -> (23.1562, 4.8822) centre (19.2671, 8.7712) ccw projected
  arc A472 (23.1562, 4.8822) -> (19.2671, 3.2712) centre (19.2671, 8.7712) ccw projected
  circle A473 centre (19.2671, 8.7712) radius 5.5 projected
  circle A474 centre (17.1458, 27.8631) radius 3 projected
  circle A475 centre (27.7524, 17.2565) radius 3 projected
  line L146 (22.4784, 40.9739) -> (13.2567, 31.7522) projected
  line L147 (13.2567, 31.7522) -> (4.7714, 23.2669) projected
  line L148 (22.4784, 40.9739) -> (4.7714, 23.2669) projected
  line L149 (23.1562, 4.8822) -> (31.6415, 13.3674) projected
  line L150 (31.6415, 13.3674) -> (40.8632, 22.5892) projected
  line L151 (23.1562, 4.8822) -> (40.8632, 22.5892) projected
  line L152 (40.8632, 22.5892) -> (22.4784, 40.9739) projected
  line L153 (40.8632, 22.5892) -> (22.4784, 40.9739) projected
  line L154 (3.1605, 19.3778) -> (3.1605, 6.1234) projected
  line L155 (3.1605, 19.3778) -> (3.1605, 6.1234) projected
  circle A476 centre (19.2671, -8.4864) radius 2.5 projected
  circle A477 centre (19.2671, -8.4864) radius 1.5 projected
  circle A478 centre (19.2671, -8.4864) radius 2.5 projected
  circle A479 centre (19.2671, -8.4864) radius 1.5 projected
  line L156 (21.0349, -31.4674) -> (24.3936, -28.1087) projected
  line L157 (17.1458, -27.5783) -> (22.4491, -22.275) projected
  line L158 (24.3936, -20.3305) -> (16.8521, -20.3305) construction
  circle A480 centre (17.1458, -27.5783) radius 2.5 projected
  circle A481 centre (17.1458, -27.5783) radius 2.5 projected
  circle A482 centre (17.1458, -27.5783) radius 2.5 projected
  line L159 (17.1458, -27.5783) -> (13.2567, -31.4674) projected
  circle A483 centre (17.1458, -27.5783) radius 3 projected
  circle A484 centre (17.1458, -27.5783) radius 5.5 projected
  circle A485 centre (17.1458, -27.5783) radius 5.5 projected
  line L160 (20.5045, -24.2196) -> (13.9798, -17.6948) projected
  line L161 (20.5045, -20.3305) -> (23.3382, -23.1642) projected
  line L162 (20.5045, -20.3305) -> (23.3382, -23.1642) projected
  line L163 (17.5046, -14.1486) -> (14.3226, -10.9666) projected
  line L164 (26.1667, -22.8107) -> (14.3226, -10.9666) projected
  line L165 (26.1667, -22.8107) -> (14.3226, -10.9666) projected
  line L166 (14.3226, -10.9666) -> (26.1667, -22.8107) projected
  line L167 (25.9899, -22.9874) -> (13.417, -10.4145) projected
  line L168 (17.5046, -14.1486) -> (26.1667, -22.8107) projected
  line L169 (12.7316, -12.5576) -> (10.4816, -12.5576) projected
  line L170 (12.7316, -12.5576) -> (10.4816, -12.5576) projected
  arc A486 (10.4816, -12.5576) -> (11.1407, -14.1486) centre (12.7316, -12.5576) ccw projected
  arc A487 (10.4816, -12.5576) -> (11.1407, -14.1486) centre (12.7316, -12.5576) ccw projected
  arc A488 (10.4816, -12.5576) -> (11.1407, -14.1486) centre (12.7316, -12.5576) ccw projected
  arc A489 (10.5886, -13.2429) -> (11.1407, -14.1486) centre (12.7316, -12.5576) ccw projected
  arc A490 (10.5886, -13.2429) -> (11.1407, -14.1486) centre (12.7316, -12.5576) ccw projected
  line L171 (12.7316, -12.5576) -> (10.4816, -12.5576) projected
  arc A491 (14.3226, -17.3306) -> (17.5046, -14.1486) centre (15.9136, -15.7396) ccw projected
  line L172 (11.1407, -14.1486) -> (14.3226, -17.3306) projected
  line L173 (12.3728, -15.3807) -> (12.5496, -15.204) projected
  line L174 (11.1407, -14.1486) -> (12.3728, -15.3807) projected
  arc A492 (14.3226, -17.3306) -> (18.0567, -15.0542) centre (15.9136, -15.7396) ccw projected
  arc A493 (14.3226, -17.3306) -> (17.5046, -14.1486) centre (15.9136, -15.7396) ccw projected
  line L175 (23.1615, -25.8159) -> (10.5886, -13.2429) projected
  line L176 (23.1615, -25.8159) -> (10.5886, -13.2429) projected
  line L177 (11.1407, -14.1486) -> (22.9847, -25.9926) projected
  line L178 (22.9847, -25.9926) -> (11.1407, -14.1486) projected
  line L179 (11.1407, -14.1486) -> (22.9847, -25.9926) projected
  line L180 (22.9847, -25.9926) -> (14.3226, -17.3306) projected
  line L181 (25.9899, -22.9874) -> (26.1667, -22.8107) projected
  line L182 (22.9847, -25.9926) -> (26.1667, -22.8107) projected
  line L183 (26.1667, -22.8107) -> (22.9847, -25.9926) projected
  line L184 (23.1615, -25.8159) -> (22.9847, -25.9926) projected
  line L185 (22.9847, -25.9926) -> (23.1615, -25.8159) projected
  line L186 (20.5045, -24.2196) -> (25.8372, -29.5522) projected
  line L187 (29.7263, -25.6631) -> (33.6153, -29.5522) projected
  line L188 (26.1667, -22.8107) -> (25.9899, -22.9874) projected
  circle A494 centre (8.6605, -19.0931) radius 2.5 projected
  circle A495 centre (8.6605, -19.0931) radius 2.5 projected
  circle A496 centre (8.6605, -19.0931) radius 5.5 projected
  circle A497 centre (8.6605, -19.0931) radius 5.5 projected
  circle A498 centre (8.6605, -19.0931) radius 3 projected
  line L189 (13.2567, -31.4674) -> (4.7714, -22.9821) projected
  line L190 (13.2567, -31.4674) -> (4.7714, -22.9821) projected
  line L191 (6.1605, -19.0931) -> (3.1605, -19.0931) projected
  line L192 (31.6415, -13.0826) -> (23.1562, -4.5974) projected
  line L193 (31.6415, -13.0826) -> (23.1562, -4.5974) projected
  circle A499 centre (0.0316, 0.1424) radius 2.5 projected
  circle A500 centre (0.0316, 0.1424) radius 2.5 projected
  circle A501 centre (0.0316, 0.1424) radius 2.5 projected
  circle A502 centre (0.0316, 0.1424) radius 2.5 projected
  circle A503 centre (0.0316, 0.1424) radius 5.5 projected
  circle A504 centre (0.0316, 0.1424) radius 6.75 projected
  line L194 (-6.9395, -3.6467) -> (-6.2792, -2.9864) projected
  line L195 (24.3936, -20.3305) -> (22.4331, -18.3699) projected
  line L196 (23.8633, -20.8608) -> (27.7524, -16.9717) projected
  circle A505 centre (27.7524, -16.9717) radius 5.5 projected
  circle A506 centre (27.7524, -16.9717) radius 5.5 projected
  circle A507 centre (27.7524, -16.9717) radius 2.5 projected
  circle A508 centre (27.7524, -16.9717) radius 2.5 projected
  circle A509 centre (27.7524, -16.9717) radius 3 projected
  line L197 (24.3936, -20.3305) -> (29.7263, -25.6631) projected
  line L198 (28.2827, -24.2196) -> (31.6415, -20.8608) projected
  line L199 (27.7524, -16.9717) -> (31.6415, -13.0826) projected
  circle A510 centre (27.7524, -16.9717) radius 2.5 projected
  circle A511 centre (19.2671, -8.4864) radius 2.5 projected
  circle A512 centre (19.2671, -8.4864) radius 2.5 projected
  circle A513 centre (19.2671, -8.4864) radius 2.5 projected
  circle A514 centre (19.2671, -8.4864) radius 5.5 projected
  line L200 (15.378, -12.3755) -> (15.9083, -11.8452) projected
  line L201 (15.5548, -12.1988) -> (15.9136, -12.5576) projected
  arc A515 (15.378, -12.3755) -> (15.569, -12.5576) centre (19.2671, -8.4864) ccw projected
  arc A516 (15.378, -12.3755) -> (15.569, -12.5576) centre (19.2671, -8.4864) ccw projected
  circle A517 centre (19.2671, -8.4864) radius 3 projected
  line L202 (6.1605, 19.3778) -> (3.1605, 19.3778) projected
  circle A518 centre (8.6605, 19.3778) radius 2.5 projected
  circle A519 centre (8.6605, 19.3778) radius 5.5 projected
  line L203 (13.2567, 31.7522) -> (4.7714, 23.2669) projected
  line L204 (31.6415, -13.0826) -> (40.8632, -22.3044) projected
  line L205 (31.6415, -13.0826) -> (40.8632, -22.3044) projected
  line L206 (33.6153, -29.5522) -> (40.8632, -22.3044) projected
  line L207 (33.6153, -29.5522) -> (40.8632, -22.3044) projected
  line L208 (-33.5521, -29.5522) -> (-29.663, -33.4413) projected
  circle A520 centre (-8.5972, -19.0931) radius 2.5 projected
  line L209 (-3.0972, -19.0931) -> (-3.0972, -12.6302) projected
  line L210 (-6.0972, -19.0931) -> (-3.0972, -19.0931) projected
  circle A521 centre (-17.0825, -27.5783) radius 2.5 projected
  circle A522 centre (-17.0825, -27.5783) radius 5.5 projected
  line L211 (-29.663, -33.4413) -> (-22.4151, -40.6891) projected
  line L212 (-13.1934, -31.4674) -> (-22.4151, -40.6891) projected
  circle A523 centre (-8.5972, -19.0931) radius 5.5 projected
  line L213 (-13.1934, -31.4674) -> (-4.7081, -22.9821) projected
  line L214 (-3.0972, -19.0931) -> (-3.0972, -12.6302) projected
  line L215 (-31.5782, -13.0826) -> (-40.7999, -22.3044) projected
  line L216 (-31.5782, -13.0826) -> (-23.0929, -4.5974) projected
  line L217 (-33.5521, -29.5522) -> (-40.7999, -22.3044) projected
  circle A524 centre (-27.6891, -16.9717) radius 2.5 projected
  circle A525 centre (-27.6891, -16.9717) radius 5.5 projected
  arc A526 (14.3226, -10.9666) -> (12.7316, -10.3076) centre (12.7316, -12.5576) ccw projected
  arc A527 (14.3226, -10.9666) -> (12.7316, -10.3076) centre (12.7316, -12.5576) ccw projected
  arc A528 (14.3226, -10.9666) -> (13.417, -10.4145) centre (12.7316, -12.5576) ccw projected
  arc A529 (14.3226, -10.9666) -> (13.417, -10.4145) centre (12.7316, -12.5576) ccw projected
  arc A530 (14.3226, -10.9666) -> (12.7316, -10.3076) centre (12.7316, -12.5576) ccw projected
  line L218 (14.3226, -10.9666) -> (14.3956, -11.0396) projected
  arc A531 (23.1562, -4.5974) -> (14.3956, -11.0396) centre (19.2671, -8.4864) ccw projected
  arc A532 (23.1562, -4.5974) -> (14.3956, -11.0396) centre (19.2671, -8.4864) ccw projected
  arc A533 (23.1562, -4.5974) -> (14.3956, -11.0396) centre (19.2671, -8.4864) ccw projected
  line L219 (14.3226, -10.9666) -> (7.0028, -3.6467) projected
  line L220 (7.0028, -3.6467) -> (6.3425, -2.9864) projected
  line L221 (19.2671, -2.9864) -> (6.0127, -2.9864) projected
  line L222 (19.2671, -2.9864) -> (6.0127, -2.9864) projected
  line L223 (19.2671, 3.2712) -> (6.0127, 3.2712) projected
  line L224 (17.4993, -10.2542) -> (23.1562, -4.5974) projected
  line L225 (12.7316, -10.3076) -> (12.7316, -12.5576) projected
  line L226 (12.7316, -10.3076) -> (12.7316, -12.5576) projected
  line L227 (12.7316, -10.3076) -> (12.7316, -12.5576) projected
  line L228 (14.3226, -10.9666) -> (3.9708, -10.9666) construction
  line L229 (3.1605, -12.6302) -> (3.1605, -5.8386) projected
  line L230 (3.1605, -12.6302) -> (3.1605, -5.8386) projected
  circle A534 centre (0.0316, -12.5576) radius 2.5 projected
  circle A535 centre (0.0316, -12.5576) radius 2.5 projected
  line L231 (-3.0972, -12.6302) -> (-3.0972, -5.8386) projected
  line L232 (-3.0972, -12.6302) -> (-3.0972, -5.8386) projected
  line L233 (0.0316, 0.1424) -> (0.0316, -12.5576) projected
  line L234 (0.0316, 0.1424) -> (12.7316, 0.1424) projected
  line L235 (0.0316, 0.1424) -> (12.7316, 0.1424) projected
  line L236 (-19.2038, -2.9864) -> (-5.9494, -2.9864) projected
  circle A536 centre (-19.2038, -8.4864) radius 2.5 projected
  circle A537 centre (-19.2038, -8.4864) radius 5.5 projected
  arc A538 (-14.3323, -11.0396) -> (-23.0929, -4.5974) centre (-19.2038, -8.4864) ccw projected
  arc A539 (-14.3323, -11.0396) -> (-23.0929, -4.5974) centre (-19.2038, -8.4864) ccw projected
  line L237 (3.1605, -19.0931) -> (3.1605, -12.6302) projected
  line L238 (3.1605, -19.0931) -> (3.1605, -12.6302) projected
  line L239 (-6.9395, 3.9315) -> (-6.2792, 3.2712) projected
  line L240 (-13.1934, 31.7522) -> (-4.7081, 23.2669) projected
  circle A540 centre (-17.0825, 27.8631) radius 2.5 projected
  circle A541 centre (-17.0825, 27.8631) radius 5.5 projected
  line L241 (-13.1934, 31.7522) -> (-22.4151, 40.9739) projected
  circle A542 centre (-27.6891, 17.2565) radius 5.5 projected
  line L242 (-31.5782, 13.3674) -> (-40.7999, 22.5892) projected
  line L243 (-29.663, 33.7261) -> (-22.4151, 40.9739) projected
  line L244 (-33.5521, 29.837) -> (-29.663, 33.7261) projected
  line L245 (-33.5521, 29.837) -> (-40.7999, 22.5892) projected
  circle A543 centre (-27.6891, 17.2565) radius 2.5 projected
  line L246 (3.1605, 19.3778) -> (3.1605, 12.915) projected
  line L247 (3.1605, 19.3778) -> (3.1605, 12.915) projected
  line L248 (-3.0972, 19.3778) -> (-3.0972, 12.915) projected
  circle A544 centre (0.0316, 12.8424) radius 2.5 projected
  circle A545 centre (0.0316, 12.8424) radius 2.5 projected
  line L249 (3.1605, 12.915) -> (3.1605, 6.1234) projected
  line L250 (3.1605, 12.915) -> (3.1605, 6.1234) projected
  line L251 (-3.0972, 12.915) -> (-3.0972, 6.1234) projected
  line L252 (0.0316, 0.1424) -> (0.0316, 12.8424) projected
  line L253 (0.0316, 0.1424) -> (0.0316, 12.8424) projected
  line L254 (-3.0972, 12.915) -> (-3.0972, 6.1234) projected
  line L255 (0.0316, 0.1424) -> (-12.6684, 0.1424) projected
  circle A546 centre (-8.5972, 19.3778) radius 2.5 projected
  circle A547 centre (-8.5972, 19.3778) radius 5.5 projected
  line L256 (-6.0972, 19.3778) -> (-3.0972, 19.3778) projected
  line L257 (-3.0972, 19.3778) -> (-3.0972, 12.915) projected
  circle A548 centre (-19.2038, 8.7712) radius 2.5 projected
  line L258 (-31.5782, 13.3674) -> (-23.0929, 4.8822) projected
  circle A549 centre (-19.2038, 8.7712) radius 5.5 projected
  arc A550 (-23.0929, 4.8822) -> (-14.3323, 11.3243) centre (-19.2038, 8.7712) ccw projected
  arc A551 (-23.0929, 4.8822) -> (-14.3323, 11.3243) centre (-19.2038, 8.7712) ccw projected
  line L259 (-19.2038, 3.2712) -> (-5.9494, 3.2712) projected
  line L260 (0.0316, 0.1424) -> (-12.6684, 0.1424) projected
  line L261 (31.6415, 13.3674) -> (23.1562, 4.8822) projected
  circle A552 centre (19.2671, 8.7712) radius 2.5 projected
  circle A553 centre (19.2671, 8.7712) radius 5.5 projected
  arc A554 (14.3956, 11.3243) -> (23.1562, 4.8822) centre (19.2671, 8.7712) ccw projected
  circle A555 centre (17.1458, 27.8631) radius 2.5 projected
  circle A556 centre (17.1458, 27.8631) radius 5.5 projected
  line L262 (13.2567, 31.7522) -> (22.4784, 40.9739) projected
  circle A557 centre (27.7524, 17.2565) radius 2.5 projected
  circle A558 centre (27.7524, 17.2565) radius 5.5 projected
  line L263 (31.6415, 13.3674) -> (40.8632, 22.5892) projected
  line L264 (33.6153, 29.837) -> (40.8632, 22.5892) projected
  line L265 (33.6153, 29.837) -> (29.7263, 33.7261) projected
  line L266 (29.7263, 33.7261) -> (22.4784, 40.9739) projected
  line L267 (13.2567, -31.4674) -> (22.4784, -40.6891) projected
  line L268 (13.2567, -31.4674) -> (22.4784, -40.6891) projected
  line L269 (25.9899, -29.7049) -> (25.8372, -29.5522) projected
  line L270 (23.3382, -23.1642) -> (31.6708, -31.4968) projected
  line L271 (29.1708, -28.9968) -> (27.2263, -30.9413) projected
  line L272 (29.7263, -33.4413) -> (25.9899, -29.7049) projected
  line L273 (27.2263, -30.9413) -> (31.1153, -27.0522) projected
  line L274 (29.7263, -33.4413) -> (22.4784, -40.6891) projected
  line L275 (29.7263, -33.4413) -> (22.4784, -40.6891) projected
  line L276 (33.6153, -29.5522) -> (29.7263, -33.4413) projected
  line L277 (33.6153, -29.5522) -> (29.7263, -33.4413) projected
  circle A559 centre (0.0316, 12.8424) radius 2.5 projected
  circle A560 centre (0.0316, 12.8424) radius 2.5 projected
  line L278 (3.1605, 19.3778) -> (3.1605, 6.1234) projected
  line L279 (3.1605, 19.3778) -> (3.1605, 6.1234) projected
  line L280 (3.1605, 19.3778) -> (3.1605, 6.1234) projected
  line L281 (3.1605, 19.3778) -> (3.1605, 12.915) projected
  line L282 (3.1605, 19.3778) -> (3.1605, 12.915) projected
  line L283 (3.1605, 19.3778) -> (3.1605, 6.1234) projected
  line L284 (3.1605, 19.3778) -> (3.1605, 6.1234) projected
  line L285 (3.1605, 19.3778) -> (3.1605, 6.1234) projected